厨房-置物架 (Autodesk Fusion 360 design; units mm, degrees)
part number: 2026-05-01-12-02-02-970
Autodesk Fusion 360 part; units mm, degrees
note: some values were not read from the file. Set by a fixed rule: which sketch regions a step uses.
sketch "草图1" plane through (0, 0, 0) normal (0, 0, 1) x (1, 0, 0)
  line L0 (-125, 60) -> (125, 60)
  line L1 (125, 60) -> (125, -60)
  line L2 (125, -60) -> (-125, -60)
  line L3 (-125, -60) -> (-125, 60)
  line L4 (-125, 60) -> (125, -60) construction
  line L5 (125, 60) -> (-125, -60) construction
  dimension "d1" = 250
  dimension "d2" = 120
  constraint horizontal L0
  constraint perpendicular L0 L1
  constraint parallel L0 L2
  constraint parallel L1 L3
  constraint coincident L4 origin
  constraint coincident L5 origin
  measures "d1" distance of L1 L3
  measures "d2" distance of L0 L2
extrude "拉伸1" add sketch "草图1" along normal blind 3 makes body 1
sketch "草图2" plane through (0, -60, 0) normal (0, -1, 0) x (1, 0, 0)
  line L0 (-125, 0) -> (125, 0)
  line L1 (125, 0) -> (125, 3)
  line L2 (125, 3) -> (-125, 3)
  line L3 (-125, 3) -> (-125, 0)
  line L4 (-125, 0) -> (125, 0)
  line L5 (125, 0) -> (125, 91.8243)
  line L6 (125, 91.8243) -> (-125, 91.8243)
  line L7 (-125, 91.8243) -> (-125, 0)
  constraint horizontal L4
  constraint vertical L5
  constraint horizontal L6
  constraint vertical L7
  constraint coincident L0.start L3.end
  constraint coincident L0.end L1.start
sketch "草图3" plane through (0, 0, 3) normal (0, 0, 1) x (-1, 0, 0)
  line L0 (125, 60) -> (-125, 60)
  line L1 (-125, 60) -> (-125, -60)
  line L2 (-125, -60) -> (125, -60)
  line L3 (125, -60) -> (125, 60)
  circle A0 centre (125, 60) radius 1.5
  dimension "d5" = 3
  constraint coincident L0.start L3.end
  measures "d5" diameter of A0
sweep "扫掠1" add profiles "草图3" path "草图2" along L5 L6 L7 L4 section 1 contours L0 L3 A0 | L0 L3 A0 separate body makes body 2
sketch "草图4" plane through (0, 0, 0) normal (1, 0, 0) x (0, 1, 0)
  line L0 (-60, 0) -> (60, 0)
  line L1 (60, 0) -> (60, 91.8243)
  line L2 (60, 91.8243) -> (-60, 91.8243)
  line L3 (-60, 91.8243) -> (-60, 0)
  line L4 (-60, 0) -> (-60, 91.8243)
  point P0 (-60, 91.8243)
  point P1 (60, 0)
  constraint horizontal L0
  constraint vertical L1
  constraint horizontal L2
  constraint vertical L3
  constraint coincident P0 L4
  constraint coincident P0 L2.end
  constraint coincident P1 L0.end
ref_plane "工作平面1" through (125, 0, 0) normal (-1, 0, 0) x (0, -1, 0)
